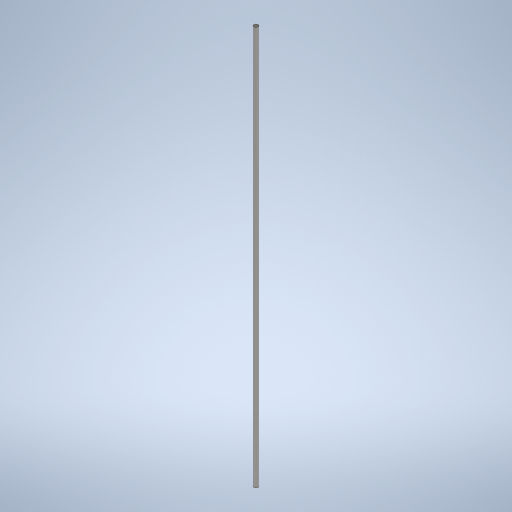
# Autodesk Inventor part: Y-belt synchronizing rod
Saved by Autodesk Inventor 2023 (Build 270158000, 158)
## iProperties
Created: 2023-02-23
Part Number: Y-belt synchronizing rod
Material: Stainless Steel
Document SubType Name: Modeling
Designer: EvanA
Density: 8 g/cm^3
Appearance: Semi-Polished
Author: EvanA
Autodesk Inventor part; units mm, degrees
ref_plane "YZ Plane" through (0, 0, 0) normal (1, 0, 0) x (0, 1, 0)
ref_plane "XZ Plane" through (0, 0, 0) normal (0, 1, 0) x (-1, 0, 0)
ref_plane "XY Plane" through (0, 0, 0) normal (0, 0, 1) x (1, 0, 0)
sketch "Sketch1" plane through (0, 0, 0) normal (0, 1, 0) x (-1, 0, 0)
  circle A0 centre (0, 0) radius 2.5
  dimension "d0" = 5
  constraints: 1 centre point, 1 coincident
  measures "d0" diameter of A0
extrude "Extrusion1" add sketch "Sketch1" along normal blind 465
chamfer "Chamfer1" distance 0.25 angle 45 2 edges at (2.5, 465, 0) (2.5, 0, 0)
body "Solid1"
